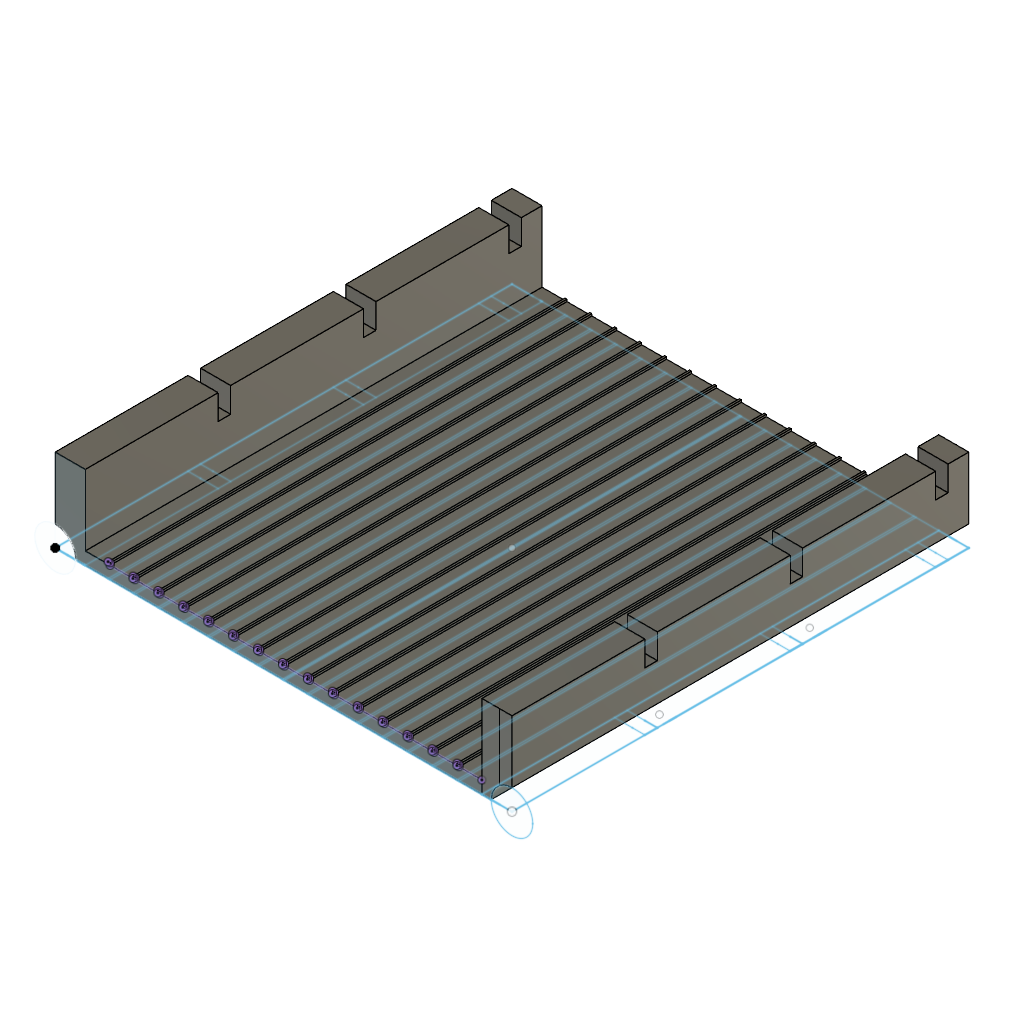
Tray_triple_EZ-Phoresis (Autodesk Fusion 360 design; units mm, degrees)
part number: 2026-01-26-09-32-51-100
Autodesk Fusion 360 part; units mm, degrees
sketch "sketch 185" plane through (0, 0, 0) normal (0, 0, 1) x (1, 0, 0)
  line L0 (255, -55) -> (145, -55)
  line L1 (145, -55) -> (145, 55)
  line L2 (145, 55) -> (255, 55)
  line L3 (255, 55) -> (255, -55)
  line L4 (145, 55) -> (150, 55)
  line L5 (150, -55) -> (145, -55)
  line L6 (145, -55) -> (145, 55)
  line L7 (255, 55) -> (250, 55)
  line L8 (250, -55) -> (255, -55)
  line L9 (255, -55) -> (255, 55)
  line L10 (255, 55) -> (255, 19)
  line L11 (255, 19) -> (255, -17)
  line L12 (200, 55) -> (200, -55)
  line L13 (255, 17.6874) -> (255, 20.6874)
  line L14 (255, -18.5) -> (255, -15.5)
  line L15 (150, -55) -> (250, -55)
  line L16 (250, -55) -> (150, -55)
  line L17 (145, -55) -> (148, -55)
  line L18 (148, -55) -> (152, -55)
  line L19 (152, -55) -> (152.25, -55)
  line L20 (152.25, -55) -> (152.25, 55)
  line L21 (152.25, 55) -> (152, 55)
  line L22 (152, -55) -> (151.75, -55)
  line L23 (151.75, 55) -> (152, 55)
  line L24 (157.75, -55) -> (157.75, 55)
  line L25 (158.25, -55) -> (158.25, 55)
  line L26 (163.75, -55) -> (163.75, 55)
  line L27 (164.25, -55) -> (164.25, 55)
  line L28 (169.75, -55) -> (169.75, 55)
  line L29 (170.25, -55) -> (170.25, 55)
  line L30 (175.75, -55) -> (175.75, 55)
  line L31 (176.25, -55) -> (176.25, 55)
  line L32 (181.75, -55) -> (181.75, 55)
  line L33 (182.25, -55) -> (182.25, 55)
  line L34 (187.75, -55) -> (187.75, 55)
  line L35 (188.25, -55) -> (188.25, 55)
  line L36 (193.75, -55) -> (193.75, 55)
  line L37 (194.25, -55) -> (194.25, 55)
  line L38 (199.75, -55) -> (199.75, 55)
  line L39 (200.25, -55) -> (200.25, 55)
  line L40 (205.75, -55) -> (205.75, 55)
  line L41 (206.25, -55) -> (206.25, 55)
  line L42 (211.75, -55) -> (211.75, 55)
  line L43 (212.25, -55) -> (212.25, 55)
  line L44 (217.75, -55) -> (217.75, 55)
  line L45 (218.25, -55) -> (218.25, 55)
  line L46 (223.75, -55) -> (223.75, 55)
  line L47 (224.25, -55) -> (224.25, 55)
  line L48 (229.75, -55) -> (229.75, 55)
  line L49 (230.25, -55) -> (230.25, 55)
  line L50 (235.75, -55) -> (235.75, 55)
  line L51 (236.25, -55) -> (236.25, 55)
  line L52 (241.75, -55) -> (241.75, 55)
  line L53 (242.25, -55) -> (242.25, 55)
  line L54 (247.75, -55) -> (247.75, 55)
  line L55 (255, 47) -> (255, 50)
  line L56 (252, 47) -> (255, 47)
  line L57 (255, 50) -> (252, 50)
  line L58 (255, 15) -> (252, 15)
  line L59 (255, -20) -> (252, -20)
  line L60 (255, 12) -> (255, 15)
  line L61 (255, 15) -> (252, 15)
  line L62 (252, 12) -> (255, 12)
  line L63 (255, -23) -> (255, -20)
  line L64 (255, -20) -> (252, -20)
  line L65 (252, -23) -> (255, -23)
  line L66 (148, 47) -> (145, 47)
  line L67 (145, 50) -> (148, 50)
  line L68 (145, 15) -> (148, 15)
  line L69 (148, 12) -> (145, 12)
  line L70 (145, -20) -> (148, -20)
  line L71 (148, -23) -> (145, -23)
  line L72 (252, 55) -> (247.75, 55)
  line L73 (247.75, -55) -> (252, -55)
  line L74 (247.75, 55) -> (247.75, -55)
  line L75 (252, 12) -> (247.75, 12)
  line L76 (252, 15) -> (247.75, 15)
  line L77 (252, -20) -> (247.75, -20)
  line L78 (252, -23) -> (247.75, -23)
  line L79 (148, -23) -> (152.25, -23)
  line L80 (148, -20) -> (152.25, -20)
  line L81 (148, 15) -> (152.25, 15)
  line L82 (148, 12) -> (152.25, 12)
  line L83 (148, 50) -> (152.25, 50)
  line L84 (148, 47) -> (152.25, 47)
  line L85 (252, 50) -> (247.75, 50)
  line L86 (252, 47) -> (247.75, 47)
  constraint coincident L54 L75.end
  constraint perpendicular L54 L75
  constraint coincident L54 L76.end
  constraint perpendicular L54 L76
  constraint coincident L54 L77.end
  constraint perpendicular L54 L77
  constraint coincident L74 L78.end
  constraint perpendicular L74 L78
  constraint coincident L20 L79.end
  constraint perpendicular L20 L79
  constraint coincident L20 L80.end
  constraint perpendicular L20 L80
  constraint coincident L20 L81.end
  constraint perpendicular L20 L81
  constraint coincident L20 L82.end
  constraint perpendicular L20 L82
  constraint coincident L20 L83.end
  constraint perpendicular L20 L83
  constraint coincident L20 L84.end
  constraint perpendicular L20 L84
  constraint coincident L54 L85.end
  constraint perpendicular L54 L85
  constraint coincident L74 L86.end
  constraint perpendicular L74 L86
extrude "Extrude1" add sketch "sketch 185" along normal blind 3 makes body 1
extrude "Extrude2" add sketch "sketch 185" along normal blind 20 separate body contours L0 L1 L5 L6 L15 L16 L17 L18 L19 L20 L22 L71 L79 | L1 L2 L4 L6 L20 L21 L23 L67 L83 | L1 L6 L20 L69 L70 L80 L82 | L1 L6 L20 L66 L68 L81 L84 makes body 2 at (145, -44.3333, 6.6667) makes body 3 at (152.25, 25.6667, 13.3333) makes body 4 at (145, -9.3333, 6.6667) makes body 5 at (147.4167, 50, 13.3333)
extrude "Extrude3" add sketch "sketch 185" along normal blind 14 contours L1 L6 L20 L70 L71 L79 L80 | L1 L6 L20 L66 L67 L83 L84 | L1 L6 L20 L68 L69 L81 L82 bodies 1 4 3 2 5
extrude "Extrude4" add sketch "sketch 185" along normal blind 20 contours L0 L3 L8 L9 L15 L16 L54 L65 L73 L74 L78 | L3 L9 L11 L14 L54 L59 L62 L64 L74 L75 L77 | L2 L3 L7 L9 L10 L54 L57 L72 L74 L85 | L3 L9 L10 L11 L13 L54 L56 L58 L61 L74 L76 L86 bodies 1
extrude "Extrude5" add sketch "sketch 185" along normal blind 14 contours L3 L9 L54 L59 L63 L64 L65 L74 L77 L78 | L3 L9 L11 L54 L58 L60 L61 L62 L74 L75 L76 | L3 L9 L10 L54 L55 L56 L57 L74 L85 L86 bodies 1
extrude "Extrude6" add sketch "sketch 185" along normal blind 3.5 contours L0 L2 L15 L16 L52 L53 | L0 L2 L15 L16 L50 L51 | L0 L2 L15 L16 L48 L49 | L0 L2 L15 L16 L46 L47 | L0 L2 L15 L16 L44 L45 | L0 L2 L15 L16 L42 L43 | L0 L2 L15 L16 L40 L41 | L0 L2 L12 L15 L16 L39 | L0 L2 L12 L15 L16 L38 | L0 L2 L15 L16 L36 L37 | L0 L2 L15 L16 L34 L35 | L0 L2 L15 L16 L32 L33 | L0 L2 L15 L16 L30 L31 | L0 L2 L15 L16 L28 L29 | L0 L2 L15 L16 L26 L27 | L0 L2 L15 L16 L24 L25 bodies 1
sketch "CircleCut" plane through (0, -55, 0) normal (0, -1, 0) x (1, 0, 0)
  line L0 (145, 0) -> (247.75, 0)
  line L1 (247.75, 0) -> (247.75, 3)
  line L2 (157.75, 3) -> (152.25, 3)
  line L3 (152.25, 3) -> (152.25, 20)
  line L4 (152.25, 20) -> (145, 20)
  line L5 (145, 20) -> (145, 0)
  circle A0 centre (145, 0) radius 5
  circle A1 centre (255, 0) radius 5
  line L6 (247.75, 3) -> (242.25, 3)
  line L7 (242.25, 3) -> (242.25, 3.5)
  line L8 (242.25, 3.5) -> (241.75, 3.5)
  line L9 (241.75, 3.5) -> (241.75, 3)
  line L10 (241.75, 3) -> (236.25, 3)
  line L11 (236.25, 3) -> (236.25, 3.5)
  line L12 (236.25, 3.5) -> (235.75, 3.5)
  line L13 (235.75, 3.5) -> (235.75, 3)
  line L14 (235.75, 3) -> (230.25, 3)
  line L15 (230.25, 3) -> (230.25, 3.5)
  line L16 (230.25, 3.5) -> (229.75, 3.5)
  line L17 (229.75, 3.5) -> (229.75, 3)
  line L18 (229.75, 3) -> (224.25, 3)
  line L19 (224.25, 3) -> (224.25, 3.5)
  line L20 (224.25, 3.5) -> (223.75, 3.5)
  line L21 (223.75, 3.5) -> (223.75, 3)
  line L22 (223.75, 3) -> (218.25, 3)
  line L23 (218.25, 3) -> (218.25, 3.5)
  line L24 (218.25, 3.5) -> (217.75, 3.5)
  line L25 (217.75, 3.5) -> (217.75, 3)
  line L26 (217.75, 3) -> (212.25, 3)
  line L27 (212.25, 3) -> (212.25, 3.5)
  line L28 (212.25, 3.5) -> (211.75, 3.5)
  line L29 (211.75, 3.5) -> (211.75, 3)
  line L30 (211.75, 3) -> (206.25, 3)
  line L31 (206.25, 3) -> (206.25, 3.5)
  line L32 (206.25, 3.5) -> (205.75, 3.5)
  line L33 (205.75, 3.5) -> (205.75, 3)
  line L34 (205.75, 3) -> (200.25, 3)
  line L35 (200.25, 3) -> (200.25, 3.5)
  line L36 (200.25, 3.5) -> (199.75, 3.5)
  line L37 (199.75, 3.5) -> (199.75, 3)
  line L38 (199.75, 3) -> (194.25, 3)
  line L39 (194.25, 3) -> (194.25, 3.5)
  line L40 (194.25, 3.5) -> (193.75, 3.5)
  line L41 (193.75, 3.5) -> (193.75, 3)
  line L42 (193.75, 3) -> (188.25, 3)
  line L43 (188.25, 3) -> (188.25, 3.5)
  line L44 (188.25, 3.5) -> (187.75, 3.5)
  line L45 (187.75, 3.5) -> (187.75, 3)
  line L46 (187.75, 3) -> (182.25, 3)
  line L47 (182.25, 3) -> (182.25, 3.5)
  line L48 (182.25, 3.5) -> (181.75, 3.5)
  line L49 (181.75, 3.5) -> (181.75, 3)
  line L50 (181.75, 3) -> (176.25, 3)
  line L51 (176.25, 3) -> (176.25, 3.5)
  line L52 (176.25, 3.5) -> (175.75, 3.5)
  line L53 (175.75, 3.5) -> (175.75, 3)
  line L54 (175.75, 3) -> (170.25, 3)
  line L55 (170.25, 3) -> (170.25, 3.5)
  line L56 (170.25, 3.5) -> (169.75, 3.5)
  line L57 (169.75, 3.5) -> (169.75, 3)
  line L58 (169.75, 3) -> (164.25, 3)
  line L59 (164.25, 3) -> (164.25, 3.5)
  line L60 (164.25, 3.5) -> (163.75, 3.5)
  line L61 (163.75, 3.5) -> (163.75, 3)
  line L62 (163.75, 3) -> (158.25, 3)
  line L63 (158.25, 3) -> (158.25, 3.5)
  line L64 (158.25, 3.5) -> (157.75, 3.5)
  line L65 (157.75, 3.5) -> (157.75, 3)
  dimension "d15" = 10
  dimension "d18" = 10
  constraint coincident L0.start L5.end
  measures "d15" diameter of A0
  measures "d18" diameter of A1
extrude "Extrude8" cut sketch "CircleCut" against normal blind 110 contours L0 L5 A0 picked at (146.1619, 3.1152) bodies 1
extrude "Extrude9" cut sketch "CircleCut" against normal blind 110 contours A1 bodies 1
named bodies: "Tray"
